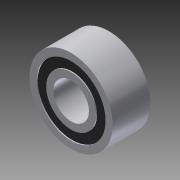
# Autodesk Inventor part: Bearing 3202 2RS - 15x35x15,9 mm
Saved by Autodesk Inventor 2013 (Build 170138000, 138)
## iProperties
Created: 2014-10-09
Part Number: Bearing 3202 2RS - 15x35x15,9 mm
Material: Generic
Document SubType Name: Modeling
Designer: Masta
Density: 1 g/cm^3
Author: Masta
Autodesk Inventor part; units mm, degrees
ref_plane "YZ Plane" through (0, 0, 0) normal (1, 0, 0) x (0, 1, 0)
ref_plane "XZ Plane" through (0, 0, 0) normal (0, 1, 0) x (-1, 0, 0)
ref_plane "XY Plane" through (0, 0, 0) normal (0, 0, 1) x (1, 0, 0)
sketch "Sketch1" plane through (0, 0, 0) normal (0, 1, 0) x (-1, 0, 0)
  circle A0 centre (0, 0) radius 7.5
  circle A1 centre (0, 0) radius 10.5
  circle A2 centre (0, 0) radius 17.5
  circle A3 centre (0, 0) radius 14.5
  dimension "d0" = 15
  dimension "d2" = 35
  dimension "d3" = 3
  dimension "d4" = 3
  constraints: 4 centre point, 4 coincident
  measures "d0" diameter of A0
  measures "d2" diameter of A2
  measures "d3" radial gap between concentric circles of A1 A0
  measures "d4" radial gap between concentric circles of A2 A3
extrude "Extrusion1" add sketch "Sketch1" along normal mid plane 15.9
extrude "Extrusion2" add sketch "Sketch1" along normal mid plane 15 contours A3
body "Solid1"
